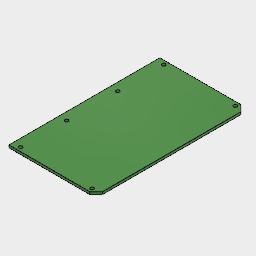
DI_card (Autodesk Fusion 360 archive; units mm, degrees)
design "PCB"
Autodesk Fusion 360 part; units mm, degrees
sketch "Sketch1" plane through (0, 0, 0) normal (0, 1, 0) x (1, 0, 0)
  line L0 (30, -47.5) -> (-30, -47.5)
  line L1 (-30, -47.5) -> (-30, 47.5)
  line L2 (-30, 47.5) -> (30, 47.5)
  line L3 (30, 47.5) -> (30, -47.5)
  line L4 (30, -47.5) -> (-30, 47.5) construction
  line L5 (-30, -47.5) -> (30, 47.5) construction
  dimension "d1" = 60
  dimension "d2" = 95
  measures "d1" distance of L0.start L0.end
  measures "d2" distance of L0.end L1.end
extrude "Extrude1" add sketch "Sketch1" along normal blind 1.6
chamfer "Chamfer1" distance 4 angle 45 2 edges at (30, 0.8, 47.5) (30, 0.8, -47.5)
sketch "Sketch2" plane through (0, 1.6, 0) normal (0, 1, 0) x (-1, 0, 0)
  line L0 (-30, -43.5) -> (-26, -47.5)
  line L1 (-26, -47.5) -> (30, -47.5)
  line L2 (30, -47.5) -> (30, 47.5)
  line L3 (30, 47.5) -> (-26, 47.5)
  line L4 (-26, 47.5) -> (-30, 43.5)
  line L5 (-30, 43.5) -> (-30, -43.5)
  line L6 (30, 0) -> (-12.828, 0) construction
  line L7 (30, -47.5) -> (25, -47.5)
  line L8 (25, -47.5) -> (25, 47.5)
  line L9 (25, 47.5) -> (30, 47.5)
  line L10 (30, 47.5) -> (30, -47.5)
  dimension "d24" = 5
  measures "d24" distance of L8.end L2.end
extrude "Extrude2" cut sketch "Sketch2" against normal through all contours L1 L2 L3 L7 L8 L9 L10
sketch "Sketch3" plane through (0, 1.6, 0) normal (0, 1, 0) x (-1, 0, 0)
  line L0 (25, 47.5) -> (-26, 47.5)
  line L1 (-26, 47.5) -> (-30, 43.5)
  line L2 (-30, 43.5) -> (-30, -43.5)
  line L3 (-30, -43.5) -> (-26, -47.5)
  line L4 (-26, -47.5) -> (25, -47.5)
  circle A0 centre (20, -45) radius 1.1
  line L5 (25, -47.5) -> (25, 47.5)
  dimension "d11" = 20
  dimension "d12" = 45
  dimension "d13" = 2.2
  measures "d11" distance of origin A0.centre
  measures "d12" distance of origin A0.centre
  measures "d13" diameter of A0
extrude "Extrude3" cut sketch "Sketch3" against normal through all contours A0
pattern_linear "R-Pattern1" count 2 spacing 45 along (1, 0, 0) count 2 spacing 90 along (0, 0, 1) of "Extrude3"
sketch "Sketch4" plane through (0, 1.6, 0) normal (0, 1, 0) x (-1, 0, 0)
  circle A0 centre (20, 45) radius 1.1
  circle A1 centre (20, -45) radius 1.1
  line L0 (25, 47.5) -> (-26, 47.5)
  line L1 (-26, 47.5) -> (-30, 43.5)
  line L2 (-30, 43.5) -> (-30, -43.5)
  line L3 (-30, -43.5) -> (-26, -47.5)
  line L4 (-26, -47.5) -> (25, -47.5)
  line L5 (20, -24) -> (20, 17) construction
  line L6 (0, 0) -> (36, 0) construction
  circle A2 centre (20, -16) radius 1.05
  circle A3 centre (20, 16) radius 1.05
  circle A4 centre (-25, 45) radius 1.1
  circle A5 centre (-25, -45) radius 1.1
  line L7 (25, -47.5) -> (25, 47.5)
  dimension "d19" = 32
  dimension "d20" = 16
  dimension "d21" = 20
  dimension "d22" = 2.1
  measures "d19" distance of A2.centre A3.centre
  measures "d20" distance of L6 A3.centre
  measures "d21" distance of L6.start L5
  measures "d22" diameter of A2
extrude "Extrude4" cut sketch "Sketch4" against normal through all contours A2 | A3
